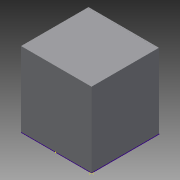
# Autodesk Inventor part: Incubation_box
Saved by Autodesk Inventor 2015 SP2 (Build 190223200, 223)
## iProperties
Created: 2016-11-10
Part Number: Incubation_box
Material: Generic
Document SubType Name: Modeling
Designer: nyc31
Density: 1 g/cm^3
Appearance: Default
Mass: 17001 g
Surface Area: 35169 cm^2
Volume: 17001 cm^3
Author: nyc31
Autodesk Inventor part; units mm, degrees
ref_plane "YZ Plane" through (0, 0, 0) normal (1, 0, 0) x (0, 1, 0)
ref_plane "XZ Plane" through (0, 0, 0) normal (0, 1, 0) x (-1, 0, 0)
ref_plane "XY Plane" through (0, 0, 0) normal (0, 0, 1) x (1, 0, 0)
sketch "Front_sketch" plane through (0, 0, 0) normal (0, 1, 0) x (-1, 0, 0)
  line L0 (280, 301) -> (-285, 301)
  line L1 (-285, 301) -> (-285, -309)
  line L2 (-285, -309) -> (280, -309)
  line L3 (280, -309) -> (280, 301)
  point P0 (0, 0)
  dimension "d0" = 565
  dimension "d1" = 610
  constraints: 8 end point, 2 parallel, 1 horizontal, 1 perpendicular
  measures "d0" distance of L2.end L1.end
  measures "d1" distance of L1.end L0.end
extrude "Extrusion1" add sketch "Front_sketch" along normal blind 10
sketch "Left_sketch" plane through (285, 0, 301) normal (1, 0, 0) x (0, 0, -1)
  line L0 (0, 0) -> (610, 0)
  line L1 (610, 0) -> (610, 550)
  line L2 (610, 550) -> (0, 550)
  line L3 (0, 550) -> (0, 0)
  point P0 (301, 0)
  constraints: 8 end point, 2 parallel, 1 horizontal, 1 perpendicular
extrude "Extrusion5" add sketch "Left_sketch" along normal blind 10 separate body
sketch "Right_sketch" plane through (-280, 0, -309) normal (-1, 0, 0) x (0, 0, 1)
  line L0 (610, 0) -> (0, 0)
  line L1 (0, 0) -> (0, 550)
  line L2 (0, 550) -> (610, 550)
  line L3 (610, 550) -> (610, 0)
  point P0 (309, 0)
  constraints: 8 end point, 2 parallel, 1 horizontal, 1 perpendicular
extrude "Extrusion6" add sketch "Right_sketch" along normal blind 10 separate body
sketch "Back_sketch" plane through (-280, 550, 301) normal (0, 1, 0) x (1, 0, 0)
  line L0 (-10, 610) -> (575, 610)
  line L1 (575, 610) -> (575, -10)
  line L2 (575, -10) -> (-10, -10)
  line L3 (-10, -10) -> (-10, 610)
  point P0 (280, 301)
  constraints: 8 end point, 2 parallel, 1 horizontal, 1 perpendicular
extrude "Extrusion7" add sketch "Back_sketch" along normal blind 10 separate body
sketch "Top_sketch" plane through (285, 0, 301) normal (0, 0, 1) x (1, 0, 0)
  line L0 (10, 0) -> (-575, 0)
  line L1 (-575, 0) -> (-575, 550)
  line L2 (-575, 550) -> (10, 550)
  line L3 (10, 550) -> (10, 0)
  point P0 (-285, 0)
  constraints: 8 end point, 2 parallel, 1 horizontal, 1 perpendicular
extrude "Extrusion8" add sketch "Top_sketch" along normal blind 10 separate body
sketch "Base_2D_sketch" plane through (285, 0, -309) normal (0, 0, -1) x (-1, 0, 0)
  line L0 (0, 10) -> (565, 10)
  line L1 (565, 10) -> (565, 550)
  line L2 (565, 550) -> (0, 550)
  line L3 (0, 550) -> (0, 10)
  line L4 (-5, 5) -> (570, 5)
  line L5 (570, 5) -> (570, 555)
  line L6 (570, 555) -> (-5, 555)
  line L7 (-5, 555) -> (-5, 5)
  line L8 (-10, 0) -> (575, 0)
  line L9 (575, 0) -> (575, 560)
  line L10 (575, 560) -> (-10, 560)
  line L11 (-10, 560) -> (-10, 0)
  point P0 (285, 0)
  constraints: 24 end point, 6 parallel, 3 horizontal, 3 perpendicular
